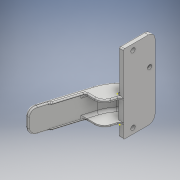
# Autodesk Inventor part: ruchka
Saved by Autodesk Inventor 2018.2 (Build 222227000, 227)
## iProperties
Created: 2026-01-25
Part Number: ruchka
Material: Типовые
Document SubType Name: Modeling
Designer: Denis
Density: 1 g/cm^3
Appearance: По умолчанию
Author: Denis
## iProperties of the stored document ruchka_3DПЕЧАТЬ.ipt
Created: 2026-01-25
Part Number: ruchka_3DПЕЧАТЬ
Material: Типовые
Document SubType Name: Modeling
Designer: Denis
Density: 1 g/cm^3
Appearance: По умолчанию
Author: Denis
Autodesk Inventor part; units mm, degrees
ref_plane "YZ Plane" through (0, 0, 0) normal (1, 0, 0) x (0, 1, 0)
ref_plane "XZ Plane" through (0, 0, 0) normal (0, 1, 0) x (-1, 0, 0)
ref_plane "XY Plane" through (0, 0, 0) normal (0, 0, 1) x (1, 0, 0)
sketch "Эскиз1" plane through (0, 0, 0) normal (0, 0, 1) x (1, 0, 0)
  line L0 (0, 0) -> (-2, 0)
  line L1 (-2, 0) -> (-5.6546, -11.9538)
  line L2 (-5.6546, -11.9538) -> (-15.1546, -11.9538)
  line L3 (-15.1546, -11.9538) -> (-25.9724, -47.3371)
  line L4 (-25.9724, -47.3371) -> (-29.3195, -46.3138)
  line L5 (-29.3195, -46.3138) -> (-14.4085, 2.4578)
  line L6 (-29.3195, -46.3138) -> (21.6805, -46.3138) construction
  line L7 (0, 0) -> (0, 26)
  line L8 (0, 26) -> (-14.4085, 2.4578)
  dimension "d0" = 2
  dimension "d1" = 12.5
  dimension "d2" = 107
  dimension "d3" = 9.5
  dimension "d4" = 37
  dimension "d5" = 3.5
  dimension "d6" = 51
  dimension "d7" = 73
  dimension "d8" = 26
  constraints: 18 end point, 2 horizontal, 2 parallel, 1 equal length, 1 perpendicular, 1 vertical
  measures "d0" distance of L0.start L0.end
  measures "d1" distance of L0.end L1.end
  measures "d2" angle of L1 L0
  measures "d3" distance of L1.end L2.end
  measures "d4" distance of L2.end L3.end
  measures "d5" distance of L3.end L4.end
  measures "d6" distance of L4.end L5.end
  measures "d7" angle of L6 L5
  measures "d8" distance of L0.start L7.end
extrude "Выдавливание1" add sketch "Эскиз1" along normal blind 20
sketch "Эскиз2" plane through (0, 0, 20) normal (0, 0, 1) x (1, 0, 0)
  line L0 (-15.1546, -11.9538) -> (-25.9724, -47.3371) projected
  line L1 (-15.1546, -11.9538) -> (-10.9159, 1.9106)
  line L2 (-29.3195, -46.3138) -> (-14.4085, 2.4578) projected
  line L3 (-10.9159, 1.9106) -> (0, 19.7927)
  line L4 (0, 0) -> (0, 26) projected
  line L5 (0, 19.7927) -> (0, -11.9538)
  line L6 (-15.1546, -11.9538) -> (-5.6546, -11.9538) projected
  line L7 (0, -11.9538) -> (-15.1546, -11.9538)
  constraints: 8 end point, 1 collinear, 1 parallel, 1 point on line, 1 vertical
extrude "Выдавливание2" cut sketch "Эскиз2" against normal blind 18
sketch "Эскиз3" plane through (0, 0, 20) normal (0, 0, 1) x (1, 0, 0)
  line L0 (-5.6546, -11.9538) -> (-15.1546, -11.9538) projected
  line L1 (-2, 0) -> (-5.6546, -11.9538) projected
  line L2 (-15.1546, -11.9538) -> (-5.6546, -11.9538)
  line L3 (0, 0) -> (-2, 0) projected
  line L4 (-5.6546, -11.9538) -> (-2, 0)
  line L5 (-2, 0) -> (0, 0)
  line L6 (0, 19.7927) -> (0, 0) projected
  line L7 (0, 0) -> (0, 19.7927)
  line L8 (-10.9159, 1.9106) -> (0, 19.7927) projected
  line L9 (0, 19.7927) -> (-10.9159, 1.9106)
  line L10 (-15.1546, -11.9538) -> (-25.9724, -47.3371) projected
  line L11 (-10.9159, 1.9106) -> (-15.1546, -11.9538)
  constraints: 12 end point, 3 collinear, 1 horizontal, 1 perpendicular
extrude "Выдавливание3" add sketch "Эскиз3" against normal blind 2
sketch "Эскиз4" plane through (0, 0, 20) normal (0, 0, 1) x (1, 0, 0)
  line L0 (0, 0) -> (0, 26) projected
  line L1 (0, 0) -> (5, 0)
  line L2 (5, 0) -> (5, 26)
  line L3 (0, 26) -> (-14.4085, 2.4578) projected
  line L4 (5, 26) -> (-14.4085, 2.4578)
  line L5 (0, 0) -> (-2, 0) projected
  line L6 (-14.4085, 2.4578) -> (0, 0)
  dimension "d15" = 5
  constraints: 8 end point, 1 horizontal, 1 perpendicular
  measures "d15" distance of L0.start L1.end
extrude "Выдавливание4" add sketch "Эскиз4" against normal blind 20 contours L6 L4 L0 | L0 L4 L2 L1
sketch "Эскиз5" plane through (0, 0, 20) normal (0, 0, 1) x (1, 0, 0)
  line L0 (5, 26) -> (0, 19.9351) projected
  line L1 (-14.4085, 2.4578) -> (-29.3195, -46.3138) projected
  line L2 (5, 26) -> (-14.4085, 2.4578)
  line L3 (-14.4085, 2.4578) -> (-2.8108, 27.723)
  line L4 (-2.8108, 27.723) -> (5, 26)
  point P0 (0, 0)
  constraints: 6 end point
extrude "Выдавливание5" cut sketch "Эскиз5" against normal blind 20
sketch "Эскиз6" plane through (0, 0, 20) normal (0, 0, 1) x (1, 0, 0)
  line L0 (-15.1546, -11.9538) -> (-5.6546, -11.9538) projected
  line L1 (-5.6546, -11.9538) -> (-0.6546, -11.9538)
  line L2 (-5.6546, -11.9538) -> (-2, 0) projected
  line L3 (-5.6546, -11.9538) -> (-2, 0)
  line L4 (-2, 0) -> (3, 0)
  line L5 (-2, 0) -> (5, 0) projected
  line L6 (3, 0) -> (-0.6546, -11.9538)
  point P0 (0, 0)
  dimension "d20" = 5
  dimension "d21" = 5
  constraints: 8 end point, 1 collinear, 1 horizontal, 1 point on line
  measures "d20" distance of L0.end L1.end
  measures "d21" distance of L2.end L4.end
extrude "Выдавливание6" add sketch "Эскиз6" against normal blind 20
sketch "Эскиз7" plane through (-0.6546, -11.9538, 20) normal (0.9563048, -0.2923717, 0) x (0, 0, -1)
  point P0 (20, 11.6229)
sketch "Эскиз8" plane through (-0.6546, -11.9538, 20) normal (0.9563048, -0.2923717, 0) x (0, 0, -1)
  line L0 (2, 10.2102) -> (2, -4.2394) projected
  line L1 (0, 12.5) -> (20, 12.5) projected
  line L2 (2, -2.0734) -> (18, -2.0734)
  line L3 (18, -2.0734) -> (18, 12.5)
  line L4 (18, 12.5) -> (2, 12.5)
  line L5 (2, 12.5) -> (2, -2.0734)
  point P0 (20, 11.6229)
  dimension "d24" = 16
  constraints: 8 end point, 2 parallel, 2 point on line, 1 horizontal, 1 perpendicular
  measures "d24" distance of L4.end L3.end
extrude "Выдавливание7" cut sketch "Эскиз8" against normal blind 6
sketch "Эскиз9" plane through (0, 0, 20) normal (0, 0, 1) x (1, 0, 0)
  line L0 (-10.93, 1.8644) -> (-15.1546, -11.9538) projected
  line L1 (-0.6546, -11.9538) -> (3, 0) projected
  line L2 (-10.93, 1.8644) -> (3, 0)
  line L3 (3, 0) -> (5, 0) projected
  line L4 (3, 0) -> (5, 0)
  line L5 (-10.93, 1.8644) -> (5, 21.0541)
  line L6 (5, 26) -> (5, 0) projected
  line L7 (5, 21.0541) -> (5, 0)
  point P0 (0, 0)
  constraints: 8 end point, 1 collinear, 1 point on line, 1 vertical
extrude "Выдавливание8" cut sketch "Эскиз9" against normal blind 18
sketch "Эскиз10" plane through (0, 0, 20) normal (0, 0, 1) x (1, 0, 0)
  line L0 (-10.93, 1.8644) -> (-15.1546, -11.9538) projected
  line L1 (-10.93, 1.8644) -> (-11.3371, 0.5328)
  line L2 (-11.3371, 0.5328) -> (2.5676, -1.4144)
  line L3 (-0.6546, -11.9538) -> (3, 0) projected
  line L4 (2.5676, -1.4144) -> (3, 0)
  line L5 (3, 0) -> (-10.93, 1.8644) projected
  line L6 (3, 0) -> (-10.93, 1.8644)
  point P0 (0, 0)
  constraints: 8 end point, 2 point on line, 1 collinear, 1 parallel
extrude "Выдавливание9" cut sketch "Эскиз10" against normal blind 18
sketch "Эскиз11" plane through (0, 0, 20) normal (0, 0, 1) x (1, 0, 0)
  line L0 (2.5676, -1.4144) -> (-11.3371, 0.5328) projected
  line L1 (3, 0) -> (-0.6546, -11.9538) projected
  line L2 (2.5676, -1.4144) -> (3, 0)
  line L3 (5, 0) -> (3, 0) projected
  line L4 (3, 0) -> (5, 0)
  line L5 (5, 21.0541) -> (5, 0) projected
  line L6 (5, 0) -> (5, 21.0541)
  line L7 (-10.93, 1.8644) -> (5, 21.0541) projected
  line L8 (5, 21.0541) -> (-10.93, 1.8644)
  line L9 (-11.3371, 0.5328) -> (-10.93, 1.8644) projected
  line L10 (-10.93, 1.8644) -> (-11.3371, 0.5328)
  line L11 (-11.3371, 0.5328) -> (2.5676, -1.4144)
  point P0 (0, 0)
  constraints: 12 end point, 5 collinear
extrude "Выдавливание10" add sketch "Эскиз11" against normal blind 2
fillet "Сопряжение1" radius 3 2 edges at (-15.1546, -11.9538, 19) (-15.1546, -11.9538, 1)
fillet "Сопряжение2" radius 8 2 edges at (-0.6546, -11.9538, 19) (-0.6546, -11.9538, 1)
fillet "Сопряжение3" radius 3 2 edges at (3, 0, 19) (3, 0, 1)
fillet "Сопряжение4" radius 30 1 edges at (-10.93, 1.8644, 10)
fillet "Сопряжение5" radius 34 1 edges at (-14.4085, 2.4578, 10)
fillet "Сопряжение6" radius 6 2 edges at (-27.6459, -46.8254, 20) (-27.6459, -46.8254, 0)
fillet "Сопряжение7" radius 2 6 edges at (-14.247, -8.9851, 2) (-1.0421, 13.7756, 2) (-10.4035, 1.5803, 2) (-1.0421, 13.7756, 18) (-14.247, -8.9851, 18) (-10.4035, 1.5803, 18)
sketch "Эскиз12" plane through (0, 0, 20) normal (0, 0, 1) x (1, 0, 0)
  point P0 (0, 0)
sketch "Эскиз13" plane through (0, 0, 20) normal (0, 0, 1) x (1, 0, 0)
  point P0 (0, 0)
sketch "Эскиз14" plane through (0, 0, 20) normal (0, 0, 1) x (1, 0, 0)
  line L0 (-15.8037, -14.0767) -> (-12.6904, -3.8936) projected
  line L1 (-14.7015, -10.4716) -> (-21.596, -33.0224)
  line L2 (-21.596, -33.0224) -> (-20.6396, -33.3147)
  line L3 (-20.6396, -33.3147) -> (-11.7341, -4.1859)
  line L4 (-12.6904, -3.8936) -> (-10.7778, -4.4783) projected
  line L5 (-12.6904, -3.8936) -> (-11.7341, -4.1859)
  point P0 (0, 0)
  dimension "d40" = 1
  dimension "d41" = 90
  constraints: 8 end point, 2 perpendicular, 2 point on line, 1 collinear, 1 midpoint
  measures "d40" distance of L1.end L2.end
  measures "d41" angle of L2 L1
extrude "Выдавливание11" add sketch "Эскиз14" against normal blind 1.2
fillet "Сопряжение8" radius 2 2 edges at (-21.596, -33.0224, 19.4) (-20.6396, -33.3147, 19.4)
fillet "Сопряжение9" radius 2 1 edges at (-14.1936, -12.2307, 19.4)
sketch "Эскиз15" plane through (0, 0, 0) normal (0, 0, -1) x (-1, 0, 0)
  arc A0 (14.5416, -13.3691) -> (12.629, -11.9538) centre (12.629, -13.9538) ccw projected
  line L0 (12.629, -11.9538) -> (35.8179, -11.9538)
  line L1 (14.5416, -13.3691) -> (20.3725, -32.441) projected
  line L2 (14.5416, -13.3691) -> (20.3725, -32.441)
  line L3 (20.3725, -32.441) -> (20.7146, -33.5599)
  arc A1 (20.3725, -32.441) -> (21.2374, -33.5599) centre (22.2851, -31.8562) ccw projected
  line L4 (20.7146, -33.5599) -> (21.6709, -33.2675)
  line L5 (15.8037, -14.0767) -> (22.1024, -34.6787) projected
  line L6 (21.6709, -33.2675) -> (14.9069, -11.1435)
  line L7 (15.8037, -14.0767) -> (12.6904, -3.8936) projected
  line L8 (14.9069, -11.1435) -> (13.9506, -11.4359)
  line L9 (13.9506, -11.4359) -> (14.5416, -13.3691)
  point P0 (0, 0)
  constraints: 14 end point, 4 point on line, 3 perpendicular, 3 tangent, 1 collinear
extrude "Выдавливание12" add sketch "Эскиз15" against normal blind 1.2 contours L9 L0 L6 L5 L4 A1 L1 | A1 L4 L3 | L9 L8 L6 L0
fillet "Сопряжение10" radius 2 3 edges at (-14.1936, -12.2307, 0.6) (-21.6709, -33.2675, 0.6) (-20.7146, -33.5599, 0.6)
sketch "Эскиз16" plane through (5, 26, 20) normal (1, 0, 0) x (0, 0, -1)
  line L0 (20, 0) -> (20, -26) projected
  line L1 (20, 0) -> (30, 0)
  line L2 (30, 0) -> (-34.3, 0)
  line L3 (-34.3, 0) -> (-34.3, -26)
  line L4 (-34.3, -26) -> (30, -26)
  line L5 (30, -26) -> (30, 0)
  dimension "d49" = 10
  dimension "d50" = 64.3
  dimension "d51" = 26
  constraints: 10 end point, 2 horizontal, 2 parallel, 1 perpendicular
  measures "d49" distance of L0.start L1.end
  measures "d50" distance of L4.end L3.end
  measures "d51" distance of L3.end L2.end
extrude "Выдавливание13" add sketch "Эскиз16" against normal blind 4
fillet "Сопряжение11" radius 10 1 edges at (1, 21.1481, 10)
fillet "Сопряжение12" radius 5.5 2 edges at (3, 26, 54.3) (3, 26, -10)
fillet "Сопряжение13" radius 1.5 4 edges at (1, 22.9434, 0) (1, 10.574, 0) (1, 10.574, 20) (1, 22.9434, 20)
sketch "Эскиз17" plane through (0, 0, 0) normal (0, 0, -1) x (-1, 0, 0)
  point P0 (0, 0)
sketch "Эскиз18" plane through (1, 26, 20) normal (-1, 0, 0) x (0, 0, 1)
  line L0 (-30, 0) -> (10.9, 0)
  line L1 (-24.5, 0) -> (28.8, 0) projected
  line L2 (10.9, 0) -> (10.9, -4.482)
  circle A0 centre (10.9, -4.482) radius 3.5
  point P0 (-20, -26)
  dimension "d57" = 40.9
  dimension "d58" = 4.482
  dimension "d59" = 7
  constraints: 4 end point, 1 centre point, 1 coincident, 1 perpendicular, 1 point on line
  measures "d57" distance of L0.start L0.end
  measures "d58" distance of L0.end L2.end
  measures "d59" diameter of A0
extrude "Выдавливание14" cut sketch "Эскиз18" against normal blind 2
sketch "Эскиз19" plane through (3, 21.518, 30.9) normal (-1, 0, 0) x (0, 0, 1)
  circle A0 centre (0, 0) radius 1.8
  point P0 (-30.9, -21.518)
  dimension "d62" = 3.6
  constraints: 1 centre point
  measures "d62" diameter of A0
extrude "Выдавливание15" cut sketch "Эскиз19" against normal blind 2
sketch "Эскиз20" plane through (1, 26, 20) normal (-1, 0, 0) x (0, 0, 1)
  line L0 (-30, 0) -> (-30, -18.182)
  line L1 (-30, -26) -> (-30, -5.5) projected
  line L2 (-30, 0) -> (-11.818, 0) construction
  line L3 (-30, -18.182) -> (-25.4, -18.182)
  circle A0 centre (-25.4, -18.182) radius 1.8
  line L4 (-25.4, -18.182) -> (29.7, -18.182)
  circle A1 centre (29.7, -18.182) radius 1.8
  point P0 (-20, -26)
  dimension "d65" = 18.182
  dimension "d66" = 90
  dimension "d67" = 4.6
  dimension "d68" = 3.6
  dimension "d69" = 55.1
  dimension "d70" = 3.6
  constraints: 8 end point, 2 centre point, 2 coincident, 2 horizontal, 2 perpendicular, 1 collinear
  measures "d65" distance of L0.start L0.end
  measures "d66" angle of L0 L2
  measures "d67" distance of L0.end L3.end
  measures "d68" diameter of A0
  measures "d69" distance of L4.start L4.end
  measures "d70" diameter of A1
extrude "Выдавливание16" cut sketch "Эскиз20" against normal blind 4
sketch "Эскиз21" plane through (1, 26, 20) normal (-1, 0, 0) x (0, 0, 1)
  point P0 (-20, -26)
fillet "Сопряжение14" radius 1 5 edges at (1, 24.3891, -8.3891) (1, 26, 22.15) (1, 24.3891, 52.6891) (1, 10.25, 54.3) (1, 10.25, -10)
fillet "Сопряжение15" radius 1 8 edges at (0.5607, 0, -0.4393) (1.2929, 0, -9.7071) (3.5, 0, -10) (1, 0, -5.25) (1.2929, 0, 54.0071) (3.5, 0, 54.3) (0.5607, 0, 20.4393) (1, 0, 37.4)
fillet "Сопряжение16" radius 2 13 edges at (-29.3195, -46.3138, 10) (-28.8057, -44.6332, 1.7574) (-21.9756, -22.2932, 0) (-13.8216, 2.1424, 0) (-5.695, 13.0271, 0) (-0.8736, 18.911, 0) (0.6434, 22.092, -0.5291) (-21.9756, -22.2932, 20) (-13.8216, 2.1424, 20) (-5.695, 13.0271, 20) (-0.8736, 18.911, 20) (0.6434, 22.092, 20.5291) (-28.8057, -44.6332, 18.2426)
fillet "Сопряжение17" radius 1 21 edges at (-23.1603, -38.139, 20) (-21.7721, -34.0403, 20) (-20.7028, -33.0794, 20) (-17.4571, -22.905, 20) (-13.8187, -12.3461, 20) (-9.6017, -11.9538, 20) (-1.8158, -10.3847, 20) (1.7148, -4.2037, 20) (3.3497, -0.648, 20) (-25.9724, -47.3371, 10) (-25.4586, -45.6565, 1.7574) (-23.1977, -38.2616, 0) (-21.847, -34.2854, 0) (-20.7777, -33.3245, 0) (-17.4945, -23.0276, 0) (-13.8187, -12.3461, 0) (-9.6017, -11.9538, 0) (-1.8158, -10.3847, 0) (1.7148, -4.2037, 0) (3.3497, -0.648, 0) (-25.4586, -45.6565, 18.2426)
